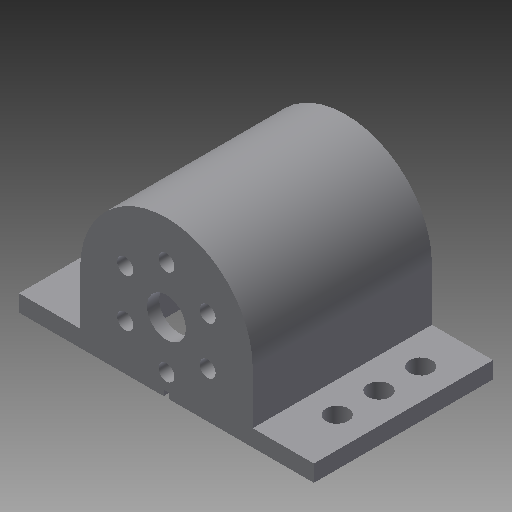
# Autodesk Inventor part: Mount gor motor TR
Saved by Autodesk Inventor 2018.1 (Build 221171000, 171)
## iProperties
Created: 2018-11-07
Part Number: Mount gor motor TR
Material: Типовые
Document SubType Name: Modeling
Designer: kostya
Density: 1 g/cm^3
Appearance: По умолчанию
Author: kostya
Autodesk Inventor part; units mm, degrees
ref_plane "YZ Plane" through (0, 0, 0) normal (1, 0, 0) x (0, 1, 0)
ref_plane "XZ Plane" through (0, 0, 0) normal (0, 1, 0) x (-1, 0, 0)
ref_plane "XY Plane" through (0, 0, 0) normal (0, 0, 1) x (1, 0, 0)
sketch "Эскиз1" plane through (0, 0, 0) normal (0, 0, 1) x (1, 0, 0)
  arc A0 (12.5, 0) -> (-12.5, 0) centre (0, 0) ccw
  line L0 (-14, -15) -> (14, 15) construction
  line L1 (14, -15) -> (-14, 15) construction
  line L2 (-14, 0) -> (14, 0) construction
  line L3 (-12.5, 0) -> (-12.5, -12.5)
  line L4 (12.5, 0) -> (12.5, -12.5)
  line L5 (-14, -12.5) -> (-12.5, -12.5)
  line L6 (12.5, -12.5) -> (14, -12.5)
  arc A1 (-12.5, 0) -> (12.5, 0) centre (0, 0) ccw construction
  line L7 (-16.5, 17.6786) -> (16.5, -17.6786) construction
  line L8 (16.5, 17.6786) -> (-16.5, -17.6786) construction
  line L9 (-16.5, -12.5) -> (-12.5, -12.5)
  line L10 (12.5, -12.5) -> (16.5, -12.5)
  arc A2 (-12.2571, 13.1326) -> (-12.5, 12.8766) centre (-1.5, 2.6786) ccw
  line L11 (16.5, -12.5) -> (26.5, -12.5)
  line L12 (0, 24.347) -> (0, -20.4254) construction
  line L13 (-16.5, -12.5) -> (-26.5, -12.5)
  line L14 (-15.5, -9.5) -> (-15.5, 0)
  arc A3 (15.5, 0) -> (-15.5, 0) centre (0, 0) ccw
  line L15 (15.5, 0) -> (15.5, -9.5)
  line L16 (-12.5, -12.5) -> (-12.5, -9.5)
  line L17 (-26.5, -12.5) -> (-12.5, -12.5)
  line L18 (-12.5, -12.5) -> (-12.5, -9.5)
  line L19 (-15.5, -9.5) -> (-26.5, -9.5)
  line L20 (-26.5, -9.5) -> (-26.5, -12.5)
  line L21 (12.5, -12.5) -> (26.5, -12.5)
  line L22 (26.5, -12.5) -> (26.5, -9.5)
  line L23 (26.5, -9.5) -> (15.5, -9.5)
  line L24 (12.5, -9.5) -> (12.5, -12.5)
  point P0 (0, 17.6786)
  dimension "d0" = 25
  dimension "d5" = 15
  dimension "d38" = 3
  dimension "d39" = 3
  constraints: 50 end point, 8 point on circle, 7 point on line, 6 perpendicular, 5 horizontal, 4 centre point, 4 midpoint, 4 parallel, 2 coincident, 2 tangent, 1 symmetric about line, 1 vertical
  measures "d0" diameter of A0
  measures "d5" radius of A2
  measures "d38" radial gap between concentric circles of A0 A3
  measures "d39" distance of L3.end L16.end
extrude "Выдавливание1" add sketch "Эскиз1" along normal mid plane 30
sketch "Эскиз7" plane through (-26.5, -9.5, 15) normal (0, 1, 0) x (1, 0, 0)
  line L0 (0, 15) -> (11, 15) construction
  line L1 (11, 30) -> (11, 0) construction
  line L2 (5.5, 0) -> (5.5, 30) construction
  line L3 (0, 30) -> (11, 30) construction
  line L4 (0, 7.5) -> (11, 7.5) construction
  line L5 (0, 22.5) -> (11, 22.5) construction
  circle A0 centre (5.5, 7.5) radius 2
  line L6 (0, 0) -> (0, 30)
  line L7 (0, 30) -> (0, 0) projected
  circle A1 centre (5.5, 15) radius 2
  circle A2 centre (5.5, 22.5) radius 2
  line L8 (26.5, 38.2442) -> (26.5, 0)
  line L9 (53, 15) -> (42, 15) construction
  line L10 (42, 30) -> (42, 0) construction
  line L11 (47.5, 0) -> (47.5, 30) construction
  line L12 (53, 30) -> (42, 30) construction
  line L13 (53, 7.5) -> (42, 7.5) construction
  line L14 (53, 22.5) -> (42, 22.5) construction
  circle A3 centre (47.5, 7.5) radius 2
  circle A4 centre (47.5, 15) radius 2
  circle A5 centre (47.5, 22.5) radius 2
  point P0 (26.5, 15)
  dimension "d40" = 4
  dimension "d41" = 4
  dimension "d42" = 4
  constraints: 24 end point, 14 symmetric about line, 6 centre point, 5 midpoint, 4 point on line, 2 perpendicular, 1 collinear, 3 other
  measures "d40" diameter of A0
  measures "d41" diameter of A1
  measures "d42" diameter of A2
extrude "Выдавливание7" cut sketch "Эскиз7" against normal blind 10
sketch "Эскиз8" plane through (0, 0, 15) normal (0, 0, 1) x (1, 0, 0)
  line L0 (-15.5, -9.5) -> (15.5, -9.5)
  constraints: 2 end point, 1 horizontal
split_face "Разделение1"
sketch "Эскиз9" plane through (0, 0, 15) normal (0, 0, 1) x (1, 0, 0)
  arc A0 (15.5, 0) -> (-15.5, 0) centre (0, 0) ccw
  line L0 (-15.5, 0) -> (-15.5, -9.5)
  line L1 (15.5, 0) -> (15.5, -9.5)
  line L2 (12.5, -12.5) -> (26.5, -12.5) projected
  line L3 (-15.5, -9.5) -> (-26.5, -9.5)
  line L4 (-26.5, -9.5) -> (-26.5, -12.5)
  line L5 (-26.5, -12.5) -> (-12.5, -12.5)
  line L6 (15.5, -9.5) -> (26.5, -9.5)
  line L7 (26.5, -9.5) -> (26.5, -12.5)
  line L8 (-12.5, -12.5) -> (12.5, -12.5)
  point P0 (-12.5, 0)
  point P1 (12.5, 0)
  point P2 (-12.5, -9.5)
  constraints: 16 end point, 3 horizontal, 2 perpendicular, 2 point on circle, 2 vertical, 1 centre point
extrude "Выдавливание8" add sketch "Эскиз9" along normal blind 2.2
sketch "Эскиз10" plane through (0, 0, 17.2) normal (0, 0, 1) x (1, 0, 0)
  arc A0 (12.5, 0) -> (-12.5, 0) centre (0, 0) ccw projected
  line L0 (12.5, 0) -> (12.5, -12.5) projected
  line L1 (-12.5, -12.5) -> (-12.5, 0) projected
  circle A1 centre (0, 0) radius 12.5 construction
  circle A2 centre (0, 0) radius 3.5
  line L2 (0, 12.5) -> (0, 10) construction
  line L3 (0, 10) -> (0, 7.1) construction
  circle A3 centre (0, 8.55) radius 1.45
  line L4 (-12.5, 0) -> (12.5, 0) construction
  circle A4 centre (-7.4045, 4.275) radius 1.45
  circle A5 centre (-7.4045, -4.275) radius 1.45
  circle A6 centre (0, -8.55) radius 1.45
  circle A7 centre (7.4045, -4.275) radius 1.45
  circle A8 centre (7.4045, 4.275) radius 1.45
  point P0 (-8.6603, 5)
  point P1 (-8.6603, -5)
  point P2 (0, -10)
  point P3 (8.6603, -5)
  point P4 (8.6603, 5)
  dimension "d47" = 7
  dimension "d48" = 2.5
  dimension "d49" = 2.9
  dimension "d52" = 360
  constraints: 6 end point, 3 vertical alignment, 2 coincident, 2 vertical, 1 centre point, 1 horizontal, 1 midpoint, 1 point on circle, 37 other
  measures "d47" diameter of A2
  measures "d48" distance of L2.start L2.end
  measures "d49" distance of L2.end L3.end
extrude "Выдавливание9" cut sketch "Эскиз10" against normal blind 3
sketch "Эскиз11" plane through (-26.5, -12.5, -15) normal (0, -1, 0) x (1, 0, 0)
  line L0 (0, 32.2) -> (53, 32.2) projected
  line L1 (26.5, 32.2) -> (26.5, 30)
  line L2 (30, 30) -> (23, 30) projected
  line L3 (27, 30) -> (26, 30)
  line L4 (26, 30) -> (26, 32.2)
  line L5 (26, 32.2) -> (27, 32.2)
  line L6 (27, 32.2) -> (27, 30)
  line L7 (27, 30) -> (26, 32.2) construction
  line L8 (26, 30) -> (27, 32.2) construction
  point P0 (26.5, 15)
  point P1 (26.5, 31.1)
  dimension "d56" = 1
  constraints: 14 end point, 5 midpoint, 2 parallel, 1 horizontal, 1 perpendicular, 1 point on line
  measures "d56" distance of L4.end L5.end
extrude "Выдавливание10" cut sketch "Эскиз11" against normal blind 1
sketch "Эскиз12" plane through (0, 0, 17.2) normal (0, 0, 1) x (1, 0, 0)
  arc A0 (15.5, 0) -> (-15.5, 0) centre (0, 0) ccw construction
  line L0 (0, 15.5) -> (0, -12.7683) construction
  constraints: 2 end point, 1 point on circle, 1 vertical
